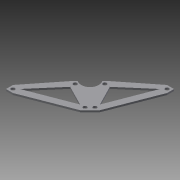
# Autodesk Inventor part: Spacer Plate
Saved by Autodesk Inventor 2013 (Build 170138000, 138)
## iProperties
Created: 2013-01-17
Part Number: Spacer Plate
Material: Generic
Document SubType Name: Modeling
Designer: actoennies
Density: 1 g/cm^3
Mass: 19.4412 g
Surface Area: 153.495 cm^2
Volume: 19.4412 cm^3
Author: actoennies
Autodesk Inventor part; units mm, degrees
ref_plane "YZ Plane" through (0, 0, 0) normal (1, 0, 0) x (0, 1, 0)
ref_plane "XZ Plane" through (0, 0, 0) normal (0, 1, 0) x (-1, 0, 0)
ref_plane "XY Plane" through (0, 0, 0) normal (0, 0, 1) x (1, 0, 0)
sketch "Sketch1" plane through (0, 0, 0) normal (0, 1, 0) x (-1, 0, 0)
  circle A0 centre (87.8158, 336.55) radius 3.3782
  circle A1 centre (0, 336.55) radius 3.3782
  circle A2 centre (95.25, 387.35) radius 3.3782
  circle A3 centre (0, 387.35) radius 3.3782
  circle A4 centre (-139.7, 0) radius 3.3782
  circle A5 centre (-103.1708, 94.1906) radius 3.3782
  circle A6 centre (-94.1906, 103.1708) radius 3.3782
  circle A7 centre (0, 139.7) radius 3.3782
  line L0 (101.6, 381) -> (101.6, 393.7)
  line L1 (101.6, 393.7) -> (90.8271, 393.7)
  line L2 (6.35, 393.7) -> (0, 393.7)
  arc A8 (0, 393.7) -> (-6.35, 393.6488) centre (0, 0) ccw
  circle A9 centre (-75.4342, 48.4934) radius 3.3782
  circle A10 centre (-48.4934, 75.4342) radius 3.3782
  line L3 (-55.6776, 55.6776) -> (-113.1015, 113.1015) construction
  line L4 (-55.6776, 55.6776) -> (-92.8744, 18.4808) construction
  line L5 (6.35, 146.05) -> (-6.35, 146.05)
  line L6 (-112.1511, 94.1906) -> (-94.1906, 112.1511)
  line L7 (-146.05, -6.35) -> (-146.05, 6.35)
  line L8 (6.35, 133.35) -> (-39.5131, 75.4342)
  line L9 (-6.35, 146.05) -> (-94.1906, 112.1511)
  line L10 (-112.1511, 94.1906) -> (-146.05, 6.35)
  line L11 (-103.1708, 85.2103) -> (-133.35, 6.35)
  line L12 (-133.35, 6.35) -> (-84.4144, 48.4934)
  line L13 (-133.35, -6.35) -> (-75.4342, 39.5131)
  line L14 (-6.35, 133.35) -> (-48.4934, 84.4144)
  line L15 (-6.35, 133.35) -> (-85.2103, 103.1708)
  line L16 (-48.4934, 84.4144) -> (-85.2103, 103.1708)
  line L17 (-84.4144, 48.4934) -> (-103.1708, 85.2103)
  line L18 (6.35, 146.05) -> (6.35, 133.35)
  line L19 (-75.4342, 39.5131) -> (-68.5543, 46.3929)
  line L20 (-46.3929, 68.5543) -> (-39.5131, 75.4342)
  line L21 (-146.05, -6.35) -> (-133.35, -6.35)
  arc A11 (-46.3929, 68.5543) -> (-68.5543, 46.3929) centre (-55.6776, 55.6776) ccw
  point P0 (-62.4128, 62.4128)
  dimension "d8" = 6.7564
  dimension "d9" = 6.7564
  dimension "d10" = 38.1
  dimension "d12" = 19.05
  dimension "d13" = 8.89
  dimension "d14" = 8.89
  dimension "d15" = 6.35
  dimension "d17" = 6.35
  dimension "d20" = 6.35
  dimension "d25" = 6.35
  dimension "d26" = 12.7
  dimension "d27" = 12.7
  dimension "d30" = 31.75
  constraints: 44 end point, 12 centre point, 4 point on circle, 2 horizontal, 2 perpendicular, 1 coincident, 1 point on line, 1 vertical, 24 other
  measures "d8" diameter of A9
  measures "d9" diameter of A10
  measures "d10" distance of A9.centre A10.centre
  measures "d12" distance from line of A9.centre L3
  measures "d13" distance from line of L4 A9.centre
  measures "d14" distance from line of L4 A10.centre
  measures "d15" distance from line of L7 A4.centre
  measures "d17" distance from line of L6 A5.centre
  measures "d20" distance from line of L5 A7.centre
  measures "d25" distance from line of L18 A7.centre
  measures "d26" distance of L14.start L5.end
  measures "d27" distance of L8.start L14.start
  measures "d30" diameter of A11
extrude "Extrusion1" add sketch "Sketch1" along normal blind 3.175 contours L18 L8 L20 A11 L19 L13 L21 L7 L10 L6 L9 L5
body "Solid1"
